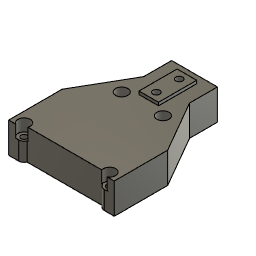
Load_Cell_Mount_v4 (Autodesk Fusion 360 design; units mm, degrees)
Autodesk Fusion 360 part; units mm, degrees
sketch "Sketch1" plane through (0, 0, 0) normal (0, 1, 0) x (1, 0, 0)
  line L0 (-7, 0) -> (-6, 0)
  line L1 (-24.7504, 0) -> (24.7504, 0)
  line L2 (-28, -2.2) -> (-34.6, -2.2)
  line L3 (28, -2.2) -> (34.6, -2.2)
  line L4 (-34.6, -2.2) -> (-34.6, 32.8)
  line L5 (-13.5, 50.8) -> (13.5, 50.8) construction
  line L6 (34.6, 32.8) -> (34.6, -2.2)
  line L7 (0, 0) -> (0, 50.8) construction
  arc A0 (-28, -2.2) -> (-24.7504, 0) centre (-28, 1.3) ccw
  arc A1 (24.7504, 0) -> (28, -2.2) centre (28, 1.3) ccw
  line L8 (15, 66.7482) -> (15, 85)
  line L9 (15, 85) -> (-15, 85)
  line L10 (-15, 85) -> (-15, 66.7482)
  circle A2 centre (-13.5, 50.8) radius 2
  circle A3 centre (13.5, 50.8) radius 2
  circle A4 centre (-28, 1.3) radius 2
  circle A5 centre (-28, 1.3) radius 4
  circle A6 centre (28, 1.3) radius 4
  circle A7 centre (28, 1.3) radius 2
  circle A8 centre (-13.5, 50.8) radius 4
  circle A9 centre (13.5, 50.8) radius 4
  line L11 (0, 85) -> (0, 50.8) construction
  line L12 (-15, 66.7482) -> (-34.6, 32.8)
  line L13 (15, 66.7482) -> (34.6, 32.8)
  line L14 (-6.4, 80) -> (6.4, 80)
  line L15 (-6.4, 80) -> (-6.4, 55)
  line L16 (-6.4, 55) -> (6.4, 55)
  line L17 (6.4, 55) -> (6.4, 80)
  circle A10 centre (0, 75) radius 2.25
  circle A11 centre (0, 60) radius 2.25
  line L18 (0, 75) -> (0, 60) construction
  line L19 (-6.4, 67.5) -> (6.4, 67.5) construction
  circle A12 centre (0, 75) radius 4.5
  circle A13 centre (0, 60) radius 4.5
  point P0 (0, 44.2)
  point P1 (0, 80)
  dimension "d10" = 6.6
  dimension "d11" = 6.6
  dimension "d12" = 35
  dimension "d13" = 35
  dimension "d14" = 49.5
  dimension "d15" = 27
  dimension "d18" = 1.3
  dimension "d19" = 1.3
  dimension "d20" = 3.5
  dimension "d21" = 3.5
  dimension "d35" = 8
  dimension "d36" = 8
  dimension "d37" = 8
  dimension "d38" = 8
  dimension "d39" = 4
  dimension "d40" = 4
  dimension "d41" = 4
  dimension "d42" = 4
  dimension "d43" = 56
  dimension "d50" = 30
  dimension "d52" = 150
  dimension "d53" = 150
  dimension "d57" = 12.8
  dimension "d58" = 25
  dimension "d59" = 15
  dimension "d60" = 4.5
  dimension "d61" = 4.5
  dimension "d62" = 80
  dimension "d63" = 5
  dimension "d66" = 9
  dimension "d67" = 9
  constraint horizontal L0
  constraint horizontal L1
  constraint tangent L2 A0
  constraint tangent L3 A1
  constraint perpendicular L2 L4
  constraint vertical L6
  constraint coincident L7.start origin
  constraint midpoint L5 L7.end
  constraint vertical L7
  constraint horizontal L5
  constraint coincident L7.start L1
  constraint vertical L4
  constraint horizontal L3
  constraint coincident L7 P0
  constraint perpendicular L8 L9
  constraint coincident L5.start A2.centre
  constraint concentric A2 A8
  constraint coincident L5.end A3.centre
  constraint concentric A3 A9
  constraint concentric A0 A4
  constraint concentric A4 A5
  constraint concentric A1 A6
  constraint concentric A6 A7
  constraint midpoint L7.start L1
  constraint midpoint L9 L11.start
  constraint vertical L11
  constraint perpendicular L11 L14
  constraint coincident L14 P1
  constraint midpoint L14 P1
  constraint coincident L11 P1
  constraint perpendicular L14 L15
  constraint perpendicular L11 L16
  constraint perpendicular L14 L17
  constraint coincident L11 A10.centre
  constraint coincident L11 A11.centre
  constraint coincident A10.centre L18.start
  constraint coincident A11.centre L18.end
  constraint midpoint L15 L19.start
  constraint midpoint L17 L19.end
  constraint midpoint L18 L19
  constraint concentric A10 A12
  constraint concentric A11 A13
  measures "d10" distance of L2.start L2.end
  measures "d11" distance of L3.start L3.end
  measures "d12" distance of L2.end L4.end
  measures "d13" distance of L3.end L6.start
  measures "d14" distance of A1.centre L5
  measures "d15" distance of L5.start L5.end
  measures "d18" distance of A0.centre L1
  measures "d19" distance of A1.centre L1
  measures "d20" radius of A0
  measures "d21" radius of A1
  measures "d35" diameter of A8
  measures "d36" diameter of A9
  measures "d37" diameter of A5
  measures "d38" diameter of A6
  measures "d39" diameter of A2
  measures "d40" diameter of A3
  measures "d41" diameter of A4
  measures "d42" diameter of A7
  measures "d43" distance of A0.centre A1.centre
  measures "d50" distance of L8 L10
  measures "d52" angle of L4 L12
  measures "d53" angle of L6 L13
  measures "d57" distance of L14.start L14.end
  measures "d58" distance of L14.end L16.end
  measures "d59" distance of A10.centre A11.centre
  measures "d60" diameter of A10
  measures "d61" diameter of A11
  measures "d62" distance of L1 L14
  measures "d63" distance of L9 L14
  measures "d66" diameter of A12
  measures "d67" diameter of A13
extrude "Extrude1" add sketch "Sketch1" along normal blind 20 contours L0 L1 L2 L3 L4 L6 L8 L9 L10 A5 A6 L12 L13 | L1 L2 A0 A5 | L1 L3 A1 A6 | A2 | A3 | A4 | A7 | A8 | A9 | L14 L15 L16 L17 | A10 | A11 | A12 | A13 picked at (-28.8891, -1.6539) picked at (28.8891, -1.6539)
extrude "Extrude2" cut sketch "Sketch1" along normal blind 20 contours A2 | A3 | A4 | A7
extrude "Extrude3" cut sketch "Sketch1" against normal blind 8 from surface at 20 contours L1 L2 A0 A5 | L1 L3 A1 A6 | A8 | A9 picked at (-28.8891, -1.6539) picked at (28.8891, -1.6539)
extrude "Extrude4" add sketch "Sketch1" along normal blind 2 from surface at 20 contours L14 L15 L16 L17 | A10 | A11 | A12 | A13
extrude "Extrude5" cut sketch "Sketch1" along normal blind 22 contours A10 | A11
extrude "Extrude6" cut sketch "Sketch1" along normal blind 4 contours A12 | A13
